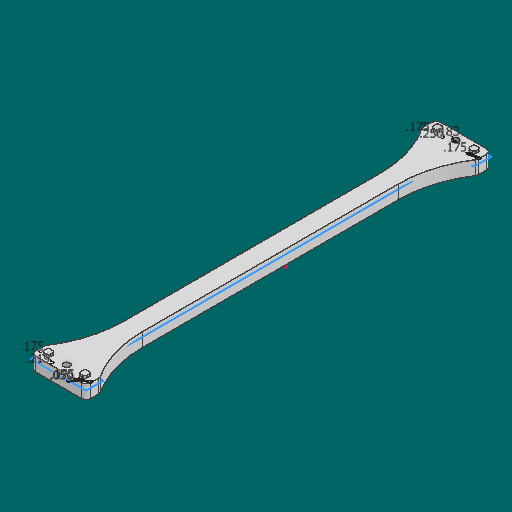
# Autodesk Inventor part: Hang_Brace
Saved by Autodesk Inventor 2025.2 (Build 292293000, 293)
## iProperties
Created: 2025-01-14
Part Number: Hang_Brace
Material: Generic
Document SubType Name: Modeling
Designer: Collin
Density: 1 g/cm^3
Appearance: Default
Author: Collin
Autodesk Inventor part; units mm, degrees
ref_plane "YZ Plane" through (0, 0, 0) normal (1, 0, 0) x (0, 1, 0)
ref_plane "XZ Plane" through (0, 0, 0) normal (0, 1, 0) x (-1, 0, 0)
ref_plane "XY Plane" through (0, 0, 0) normal (0, 0, 1) x (1, 0, 0)
sketch "Sketch1" plane through (0, 0, 0) normal (0, 1, 0) x (-1, 0, 0)
  line L0 (-5.0003, -137.0588) -> (32.1599, -137.0588)
  circle A0 centre (26.7497, 138.347) radius 2.2225
  circle A1 centre (26.7497, -131.5026) radius 2.2225
  line L1 (32.1599, -137.0588) -> (33.0997, -137.0588)
  line L2 (33.0997, -137.0588) -> (33.0997, -131.5026)
  line L3 (33.0997, 138.347) -> (33.0997, 143.9033)
  line L4 (33.0997, 143.9033) -> (-5.0003, 143.9033)
  circle A2 centre (14.0497, 138.347) radius 2.3241
  circle A3 centre (14.0497, -131.5026) radius 2.3241
  circle A4 centre (1.3497, -131.5026) radius 2.2225
  circle A5 centre (1.3497, 138.347) radius 2.2225
  line L5 (-5.0003, 143.9033) -> (-5.0003, 131.997)
  line L6 (-5.0003, -125.1526) -> (-5.0003, -137.0588)
  line L7 (33.0997, -131.5026) -> (33.0997, -125.1526)
  line L8 (33.0997, 131.997) -> (33.0997, 138.347)
  line L9 (27.7022, -129.2801) -> (25.7972, -129.2801)
  line L10 (24.5272, -130.5501) -> (24.5272, -132.4551)
  line L11 (25.7972, -133.7251) -> (27.7022, -133.7251)
  line L12 (28.9722, -132.4551) -> (28.9722, -130.5501)
  line L13 (2.3022, -129.2801) -> (0.3972, -129.2801)
  line L14 (-0.8728, -130.5501) -> (-0.8728, -132.4551)
  line L15 (0.3972, -133.7251) -> (2.3022, -133.7251)
  line L16 (3.5722, -132.4551) -> (3.5722, -130.5501)
  line L17 (27.7022, 140.5695) -> (25.7972, 140.5695)
  line L18 (24.5272, 139.2995) -> (24.5272, 137.3945)
  line L19 (25.7972, 136.1245) -> (27.7022, 136.1245)
  line L20 (28.9722, 137.3945) -> (28.9722, 139.2995)
  line L21 (2.3022, 140.5695) -> (0.3972, 140.5695)
  line L22 (-0.8728, 139.2995) -> (-0.8728, 137.3945)
  line L23 (0.3972, 136.1245) -> (2.3022, 136.1245)
  line L24 (3.5722, 137.3945) -> (3.5722, 139.2995)
  arc A6 (3.5722, 139.2995) -> (2.3022, 140.5695) centre (2.3022, 139.2995) ccw
  arc A7 (2.3022, 136.1245) -> (3.5722, 137.3945) centre (2.3022, 137.3945) ccw
  arc A8 (-0.8728, 137.3945) -> (0.3972, 136.1245) centre (0.3972, 137.3945) ccw
  arc A9 (0.3972, 140.5695) -> (-0.8728, 139.2995) centre (0.3972, 139.2995) ccw
  arc A10 (28.9722, 139.2995) -> (27.7022, 140.5695) centre (27.7022, 139.2995) ccw
  arc A11 (27.7022, 136.1245) -> (28.9722, 137.3945) centre (27.7022, 137.3945) ccw
  arc A12 (24.5272, 137.3945) -> (25.7972, 136.1245) centre (25.7972, 137.3945) ccw
  arc A13 (25.7972, 140.5695) -> (24.5272, 139.2995) centre (25.7972, 139.2995) ccw
  arc A14 (27.7022, -133.7251) -> (28.9722, -132.4551) centre (27.7022, -132.4551) ccw
  arc A15 (28.9722, -130.5501) -> (27.7022, -129.2801) centre (27.7022, -130.5501) ccw
  arc A16 (25.7972, -129.2801) -> (24.5272, -130.5501) centre (25.7972, -130.5501) ccw
  arc A17 (24.5272, -132.4551) -> (25.7972, -133.7251) centre (25.7972, -132.4551) ccw
  arc A18 (3.5722, -130.5501) -> (2.3022, -129.2801) centre (2.3022, -130.5501) ccw
  arc A19 (2.3022, -133.7251) -> (3.5722, -132.4551) centre (2.3022, -132.4551) ccw
  arc A20 (0.3972, -129.2801) -> (-0.8728, -130.5501) centre (0.3972, -130.5501) ccw
  arc A21 (-0.8728, -132.4551) -> (0.3972, -133.7251) centre (0.3972, -132.4551) ccw
  line L25 (7.6997, 131.997) -> (7.6997, -125.1526)
  line L26 (20.3997, -125.1526) -> (20.3997, 131.997)
  line L27 (14.0497, 136.1245) -> (14.0497, 136.0229)
  line L28 (14.0497, -129.1785) -> (14.0497, -129.2801)
  line L29 (-5.0003, -125.1526) -> (7.6997, -125.1526)
  line L30 (20.3997, -125.1526) -> (33.0997, -125.1526)
  line L31 (33.0997, 131.997) -> (20.3997, 131.997)
  line L32 (7.6997, 131.997) -> (-5.0003, 131.997)
  point P0 (0, 0)
  dimension "d6" = 4.6482
  dimension "d0" = 4.445
  dimension "d1" = 4.445
  dimension "d2" = 6.35
  dimension "d4" = 5.5563
  dimension "d7" = 4.445
  dimension "d8" = 4.445
  dimension "d10" = 1.27
  constraints: 66 end point, 32 point on circle, 32 tangent, 20 centre point, 15 equal radius, 12 perpendicular, 9 parallel, 5 horizontal, 3 vertical, 2 point on line, 2 vertical alignment, 4 other
  measures "d0" diameter of A0
  measures "d1" diameter of A1
  measures "d2" distance of A1.centre L2.end
  measures "d4" distance of L3.start L3.end
  measures "d7" diameter of A4
  measures "d8" diameter of A5
  measures "d10" radius of A6
extrude "Extrusion1" add sketch "Sketch1" along normal blind 3.175
extrude "Extrusion2" add sketch "Sketch1" along normal blind 4.7752 contours A0 | L20 A11 L19 A0 | A0 L17 A10 L20 | A0 L18 A13 L17 | L19 A12 L18 A0 | A1 | L12 A14 L11 A1 | A1 L9 A15 L12 | A1 L10 A16 L9 | L11 A17 L10 A1 | A4 | L16 A19 L15 A4 | A4 L13 A18 L16 | A4 L14 A20 L13 | L15 A21 L14 A4 | A5 | L24 A7 L23 A5 | A5 L21 A6 L24 | A5 L22 A9 L21 | L23 A8 L22 A5
fillet "Fillet1" radius 3.175 8 edges at (5.0003, 1.5875, -137.0588) (5.0003, 1.5875, -125.1526) (-33.0997, 1.5875, -125.1526) (-33.0997, 1.5875, -137.0588) (-33.0997, 1.5875, 131.997) (-33.0997, 1.5875, 143.9033) (5.0003, 1.5875, 143.9033) (5.0003, 1.5875, 131.997)
fillet "Fillet2" radius 76.2 4 edges at (-7.6997, 1.5875, 131.997) (-20.3997, 1.5875, 131.997) (-7.6997, 1.5875, -125.1526) (-20.3997, 1.5875, -125.1526)
sketch "Sketch2" plane through (0, 0, 0) normal (0, -1, 0) x (1, 0, 0)
  arc A0 (-20.3997, 92.1042) -> (-32.5917, 133.4493) centre (-96.5997, 92.1042) ccw projected
  arc A1 (4.4923, 133.4493) -> (-7.6997, 92.1042) centre (68.5003, 92.1042) ccw projected
  arc A2 (-32.5917, -126.6049) -> (-20.3997, -85.2598) centre (-96.5997, -85.2598) ccw projected
  arc A3 (-7.6997, -85.2598) -> (4.4923, -126.6049) centre (68.5003, -85.2598) ccw projected
  arc A4 (4.4923, 133.4493) -> (5.0003, 135.172) centre (1.8253, 135.172) ccw projected
  line L0 (5.0003, 140.7283) -> (5.0003, 135.172) projected
  arc A5 (5.0003, 140.7283) -> (1.8253, 143.9033) centre (1.8253, 140.7283) ccw projected
  line L1 (-29.9247, 143.9033) -> (1.8253, 143.9033) projected
  arc A6 (-29.9247, 143.9033) -> (-33.0997, 140.7283) centre (-29.9247, 140.7283) ccw projected
  line L2 (-33.0997, 135.172) -> (-33.0997, 140.7283) projected
  arc A7 (-33.0997, 135.172) -> (-32.5917, 133.4493) centre (-29.9247, 135.172) ccw projected
  arc A8 (-20.3997, 92.1042) -> (-32.5917, 133.4493) centre (-96.5997, 92.1042) ccw projected
  line L3 (-20.3997, -85.2598) -> (-20.3997, 92.1042) projected
  arc A9 (-32.5917, -126.6049) -> (-20.3997, -85.2598) centre (-96.5997, -85.2598) ccw projected
  arc A10 (-32.5917, -126.6049) -> (-33.0997, -128.3276) centre (-29.9247, -128.3276) ccw projected
  line L4 (-33.0997, -133.8838) -> (-33.0997, -128.3276) projected
  arc A11 (-33.0997, -133.8838) -> (-29.9247, -137.0588) centre (-29.9247, -133.8838) ccw projected
  line L5 (1.8253, -137.0588) -> (-29.9247, -137.0588) projected
  arc A12 (1.8253, -137.0588) -> (5.0003, -133.8838) centre (1.8253, -133.8838) ccw projected
  line L6 (5.0003, -128.3276) -> (5.0003, -133.8838) projected
  arc A13 (5.0003, -128.3276) -> (4.4923, -126.6049) centre (1.8253, -128.3276) ccw projected
  arc A14 (-7.6997, -85.2598) -> (4.4923, -126.6049) centre (68.5003, -85.2598) ccw projected
  line L7 (-7.6997, 92.1042) -> (-7.6997, -85.2598) projected
  arc A15 (4.4923, 133.4493) -> (-7.6997, 92.1042) centre (68.5003, 92.1042) ccw projected
  circle A16 centre (-14.0497, 138.347) radius 2.3241 projected
  circle A17 centre (-14.0497, -131.5026) radius 2.3241 projected
  point P0 (0, 0)
  point P1 (4.4923, 133.4493)
  point P2 (-32.5917, 133.4493)
  point P3 (-20.3997, 92.1042)
  point P4 (-20.3997, -85.2598)
  point P5 (-32.5917, -126.6049)
  point P6 (4.4923, -126.6049)
  point P7 (-7.6997, -85.2598)
extrude "Extrusion3" add sketch "Sketch2" along normal blind 6.35
body "Solid1"
